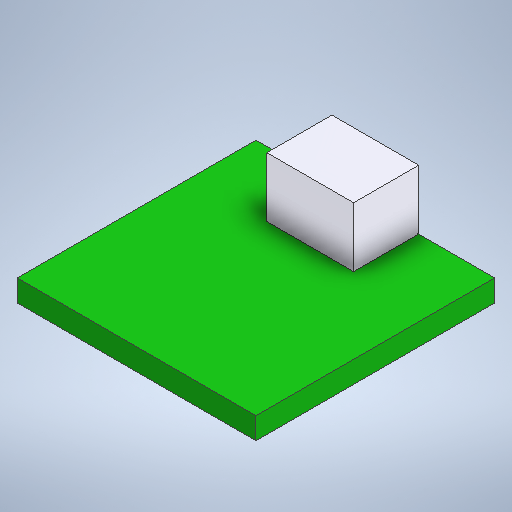
# Autodesk Inventor part: battery connector
Saved by Autodesk Inventor 2025.2 (Build 292293000, 293)
## iProperties
Created: 2025-04-04
Part Number: battery connector
Material: Generic
Document SubType Name: Modeling
Designer: joaki
Density: 1 g/cm^3
Appearance: Default
Author: joaki
Autodesk Inventor part; units mm, degrees
ref_plane "YZ Plane" through (0, 0, 0) normal (1, 0, 0) x (0, 1, 0)
ref_plane "XZ Plane" through (0, 0, 0) normal (0, 1, 0) x (-1, 0, 0)
ref_plane "XY Plane" through (0, 0, 0) normal (0, 0, 1) x (1, 0, 0)
sketch "Sketch1" plane through (0, 0, 0) normal (0, 1, 0) x (-1, 0, 0)
  line L0 (16.6199, 13.3988) -> (-5.3801, 13.3988)
  line L1 (-5.3801, 13.3988) -> (-5.3801, -8.6012)
  line L2 (-5.3801, -8.6012) -> (16.6199, -8.6012)
  line L3 (16.6199, -8.6012) -> (16.6199, 13.3988)
  point P0 (0, 0)
  dimension "d0" = 22
  dimension "d1" = 22
  constraints: 8 end point, 2 parallel, 1 horizontal, 1 perpendicular
  measures "d0" distance of L1.end L2.end
  measures "d1" distance of L0.end L1.end
extrude "Extrusion1" add sketch "Sketch1" along normal blind 2
sketch "Sketch2" plane through (0, 2, 0) normal (0, 1, 0) x (1, 0, 0)
  line L0 (5.3801, 8.6012) -> (-16.6199, 8.6012) projected
  line L1 (-1.6199, 8.6012) -> (-9.6199, 8.6012)
  line L2 (-9.6199, 8.6012) -> (-9.6199, 2.6012)
  line L3 (-9.6199, 2.6012) -> (-1.6199, 2.6012)
  line L4 (-1.6199, 2.6012) -> (-1.6199, 8.6012)
  line L5 (-16.6199, 8.6012) -> (-16.6199, -13.3988) projected
  line L6 (5.3801, -13.3988) -> (5.3801, 8.6012) projected
  point P0 (0, 0)
  dimension "d4" = 8
  dimension "d5" = 7
  dimension "d6" = 7
  dimension "d7" = 6
  constraints: 8 end point, 2 parallel, 1 horizontal, 1 perpendicular, 1 point on line
  measures "d4" distance of L2.end L3.end
  measures "d5" distance between parallel lines of L5 L2
  measures "d6" distance between parallel lines of L4 L6
  measures "d7" distance of L1.end L2.end
extrude "Extrusion2" add sketch "Sketch2" along normal blind 5.5
sketch "Sketch3" plane through (5.3801, 0, -8.6012) normal (0, 0, -1) x (-1, 0, 0)
  line L0 (7, 2) -> (15, 2) projected
  line L1 (15, 2) -> (15, 7.5) projected
  line L2 (7, 2) -> (15, 2)
  line L3 (15, 2) -> (15, 2.1)
  line L4 (15, 2.1) -> (7, 2.1)
  line L5 (7, 2.1) -> (7, 2)
  point P0 (5.3801, 0)
  dimension "d10" = 0.1
  constraints: 8 end point, 2 parallel, 1 horizontal, 1 perpendicular, 1 point on line
  measures "d10" distance between parallel lines of L4 L0
extrude "Extrusion3" cut sketch "Sketch3" against normal blind 0.1
body "Solid1"
